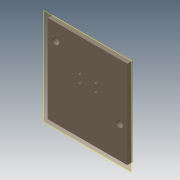
# Autodesk Inventor part: HbSensorBoard01
Saved by Autodesk Inventor 2015 SP1 (Build 190203100, 203)
## iProperties
Created: 2015-05-21
Part Number: HbSensorBoard01
Material: Generic
Document SubType Name: Modeling
Designer: Yamaura
Density: 1 g/cm^3
Appearance: Default
Author: Yamaura
Autodesk Inventor part; units mm, degrees
ref_plane "YZ Plane" through (0, 0, 0) normal (1, 0, 0) x (0, 1, 0)
ref_plane "XZ Plane" through (0, 0, 0) normal (0, 1, 0) x (-1, 0, 0)
ref_plane "XY Plane" through (0, 0, 0) normal (0, 0, 1) x (1, 0, 0)
ref_plane "作業平面1" through (0, 0, 0) normal (0, 0, 1) x (1, 0, 0)
sketch "スケッチ1" plane through (0, 0, 0) normal (0, 0, 1) x (1, 0, 0)
  line L0 (-12.7, 11.83) -> (-12.7, 13.57) projected
  line L1 (-12.3, 13.97) -> (-10.56, 13.97) projected
  line L2 (12.3, -13.97) -> (10.56, -13.97) projected
  line L3 (12.7, -11.83) -> (12.7, -13.57) projected
  line L4 (-12.7, 13.97) -> (12.7, 13.97)
  line L5 (12.7, 13.97) -> (12.7, -13.97)
  line L6 (12.7, -13.97) -> (-12.7, -13.97)
  line L7 (-12.7, -13.97) -> (-12.7, 13.97)
  point P0 (0, 0)
  constraints: 8 end point, 2 parallel, 1 horizontal, 1 perpendicular, 1 point on line
extrude "押し出し1" add sketch "スケッチ1" against normal blind 1.6
sketch "スケッチ2" plane through (0, 0, 0) normal (0, 0, 1) x (1, 0, 0)
  circle A0 centre (-10.16, 8.89) radius 1.1
  circle A1 centre (10.16, -3.81) radius 1.1
  point P0 (0, 0)
  dimension "d2" = 2.2
  dimension "d3" = 2.2
  dimension "d4" = 10.16
  dimension "d5" = 8.89
  dimension "d6" = 3.81
  dimension "d7" = 10.16
  constraints: 2 centre point
  measures "d2" diameter of A0
  measures "d3" diameter of A1
  measures "d4" horizontal distance of point (0, 0) A0.centre
  measures "d5" vertical distance of point (0, 0) A0.centre
  measures "d6" vertical distance of A1.centre point (0, 0)
  measures "d7" horizontal distance of A1.centre point (0, 0)
extrude "押し出し2" cut sketch "スケッチ2" along normal mid plane 20
sketch "スケッチ3" plane through (0, 0, 0) normal (0, 0, 1) x (1, 0, 0)
  circle A0 centre (-2.54, 3.81) radius 0.4 projected
  circle A1 centre (-2.54, 1.27) radius 0.4 projected
  circle A2 centre (2.54, 3.81) radius 0.4 projected
  circle A3 centre (2.54, 1.27) radius 0.4 projected
  point P0 (0, 0)
extrude "押し出し3" cut sketch "スケッチ3" along normal mid plane 20
sketch "スケッチ4" plane through (0, 0, 0) normal (0, 0, 1) x (1, 0, 0)
  circle A0 centre (-2.54, 1.27) radius 0.4 projected
  circle A1 centre (-2.54, 3.81) radius 0.4 projected
  circle A2 centre (2.54, 1.27) radius 0.4 projected
  circle A3 centre (2.54, 3.81) radius 0.4 projected
  circle A4 centre (0, 2.54) radius 0.05
  line L0 (0, -30.1689) -> (0, 24.3248)
  point P0 (0, 0)
  dimension "d12" = 0.1
  dimension "d13" = 2.54
  constraints: 2 end point, 1 centre point, 1 coincident, 1 point on line, 1 vertical, 2 other
  measures "d12" diameter of A4
  measures "d13" distance of point (0, 2.54) point (0, 0)
extrude "押し出し4" cut sketch "スケッチ4" against normal blind 20 contours A4 L0 | L0 A4
sketch "スケッチ5" plane through (0, 0, 0) normal (0, 0, 1) x (1, 0, 0)
  circle A0 centre (0, -3) radius 0.8
  circle A1 centre (0, -10) radius 0.8
  point P0 (0, 0)
  dimension "d16" = 1.6
  dimension "d17" = 1.6
  dimension "d18" = 3
  dimension "d19" = 7
  constraints: 2 centre point
  measures "d16" diameter of A0
  measures "d17" diameter of A1
  measures "d18" distance of A0.centre point (0, 0)
  measures "d19" distance of A1.centre A0.centre
extrude "押し出し5" cut sketch "スケッチ5" against normal blind 20
